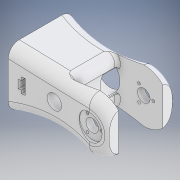
# Autodesk Inventor part: AA010
Saved by Autodesk Inventor 2017 SP1 (Build 210196100, 196)
## iProperties
Created: 2017-09-29
Part Number: AA010
Material: ABS Plastic
Document SubType Name: Modeling
Designer: Zach
Density: 1.06 g/cm^3
Appearance: CR White
Author: Zach
Autodesk Inventor part; units mm, degrees
sketch "Sketch1" plane through (0, 0, 0) normal (0, 0, 1) x (1, 0, 0)
  line L0 (0, 0) -> (0, 105)
  circle A0 centre (75, 52.5) radius 2.5
  circle A1 centre (145, 52.5) radius 11.25
  circle A2 centre (145, 52.5) radius 47.5 construction
  arc A3 (145, 5) -> (0, 0) centre (84.2999, -339.6962) ccw
  arc A4 (0, 105) -> (145, 100) centre (84.2999, 444.6962) ccw
  arc A5 (145, 5) -> (145, 100) centre (145, 52.5) ccw
  point P0 (0, 52.5)
  dimension "d0" = 105
  dimension "d1" = 5
  dimension "d2" = 22.5
  dimension "d3" = 70
  dimension "d4" = 95
  dimension "d5" = 145
  dimension "d6" = 350
  dimension "d7" = 350
  constraints: 8 point on circle, 6 centre point, 2 end point, 2 horizontal alignment, 2 vertical alignment, 1 coincident, 1 concentric, 1 midpoint, 1 vertical
  measures "d0" distance of L0.start L0.end
  measures "d1" diameter of A0
  measures "d2" diameter of A1
  measures "d3" distance of A1.centre A0.centre
  measures "d4" diameter of A2
  measures "d5" distance of point (0, 52.5) A2.centre
  measures "d6" radius of A3
  measures "d7" radius of A4
extrude "Extrusion1" add sketch "Sketch1" along normal blind 115
sketch "Sketch2" plane through (0, 0, 0) normal (0, 1, 0) x (-1, 0, 0)
  line L0 (0, 0) -> (-145, 0) projected
  arc A0 (0, 0) -> (-145, 0) centre (-72.5, -342.4087) ccw
  line L1 (-145, 115) -> (0, 115) projected
  arc A1 (-145, 115) -> (0, 115) centre (-72.5, 457.4087) ccw
  dimension "d10" = 350
  dimension "d11" = 350
  constraints: 4 point on circle, 2 centre point
  measures "d10" radius of A0
  measures "d11" radius of A1
extrude "Extrusion2" cut sketch "Sketch2" along normal through all
ref_plane "Work Plane1" through (0, 0, 57.5) normal (0, 0, 1) x (1, 0, 0)
sketch "Sketch3" plane through (0, 0, 57.5) normal (0, 0, 1) x (1, 0, 0)
  arc A0 (145, 41.25) -> (145, 63.75) centre (145, 52.5) ccw projected
  arc A1 (145, 41.25) -> (145, 63.75) centre (145, 52.5) ccw projected
  circle A2 centre (145, 52.5) radius 52.5
  point P0 (0, 0)
  dimension "d15" = 105
  constraints: 1 centre point, 1 coincident
  measures "d15" diameter of A2
extrude "Extrusion3" cut sketch "Sketch3" along normal mid plane 79
fillet "Fillet2" radius 15 2 edges at (115.7763, 96.1145, 57.5) (115.7763, 8.8855, 57.5)
fillet "Fillet3" radius 20 4 edges at (71.9844, 94.913, 7.5909) (71.9844, 94.913, 107.4091) (71.9843, 10.087, 107.4091) (71.9843, 10.087, 7.5909)
fillet "Fillet4" radius 20 2 edges at (192.5, 52.5, 115) (192.5, 52.5, 0)
sketch "Sketch4" plane through (0, 19.5779, 115) normal (-1, 0, 0) x (0, 0, 1)
  line L0 (-72, 12.9221) -> (-97, 12.9221)
  line L1 (-97, 12.9221) -> (-97, 52.9221)
  line L2 (-97, 52.9221) -> (-72, 52.9221)
  line L3 (-72, 52.9221) -> (-72, 12.9221)
  line L4 (-95.5772, -19.5779) -> (-19.4228, -19.5779) projected
  line L5 (-115, 0) -> (-115, 65.8443) projected
  line L6 (-97, -14.5765) -> (-97, -7.145) projected
  line L7 (-97, 80.4208) -> (-97, -14.5765) projected
  line L8 (-97, 72.9893) -> (-97, 80.4208) projected
  line L9 (-97, 54.076) -> (-97, 72.9893) projected
  line L10 (-97, 11.7683) -> (-97, 54.076) projected
  line L11 (-97, -7.145) -> (-97, 11.7683) projected
  line L12 (-97, 21.6721) -> (-97, 44.1721) projected
  line L13 (-18, 44.1721) -> (-18, 21.6721) projected
  line L14 (-18, -7.145) -> (-18, -14.5765) projected
  line L15 (-18, 11.7683) -> (-18, -7.145) projected
  line L16 (-18, 54.076) -> (-18, 11.7683) projected
  line L17 (-18, 72.9893) -> (-18, 54.076) projected
  line L18 (-18, 80.4208) -> (-18, 72.9893) projected
  line L19 (-18, -14.5765) -> (-18, 80.4208) projected
  point P0 (-115, -19.5779)
  point P1 (-84.5, 12.9221)
  point P2 (-57.5, -19.5779)
  point P3 (-97, 32.9221)
  point P4 (-115, 32.9221)
  dimension "d21" = 25
  dimension "d22" = 40
  constraints: 8 end point, 5 midpoint, 2 parallel, 1 horizontal, 1 horizontal alignment, 1 perpendicular
  measures "d21" distance of L1.end L2.end
  measures "d22" distance of L0.end L1.end
extrude "Extrusion4" cut sketch "Sketch4" against normal through all
sketch "Sketch6" plane through (0, 0, 0) normal (0, 0, -1) x (-1, 0, 0)
  circle A0 centre (-145, 52.5) radius 22.5
  arc A1 (-145, 63.75) -> (-145, 41.25) centre (-145, 52.5) ccw projected
  point P0 (0, 0)
  dimension "d28" = 45
  constraints: 1 centre point, 1 concentric
  measures "d28" diameter of A0
extrude "Extrusion6" cut sketch "Sketch6" against normal blind 5
sketch "Sketch7" plane through (0, 0, 115) normal (0, 0, 1) x (1, 0, 0)
  circle A0 centre (145, 52.5) radius 22.5
  arc A1 (145, 41.25) -> (145, 63.75) centre (145, 52.5) ccw projected
  point P0 (0, 0)
  dimension "d31" = 45
  constraints: 1 centre point, 1 concentric
  measures "d31" diameter of A0
extrude "Extrusion7" cut sketch "Sketch7" against normal blind 5
sketch "Sketch8" plane through (145, 52.5, 110) normal (0, 0, 1) x (1, 0, 0)
  circle A0 centre (17, 0) radius 2.5
  circle A1 centre (0, 0) radius 11.25 construction
  circle A2 centre (-8.5, 14.7224) radius 2.5
  circle A3 centre (-8.5, -14.7224) radius 2.5
  point P0 (-145, -52.5)
  dimension "d34" = 5
  dimension "d35" = 17
  dimension "d38" = 360
  constraints: 3 centre point, 1 horizontal alignment, 7 other
  measures "d34" diameter of A0
  measures "d35" distance of A0.centre A1.centre
extrude "Extrusion8" cut sketch "Sketch8" against normal through all
sketch "Sketch47" plane through (0, 0, 18) normal (0, 0, 1) x (1, 0, 0)
  circle A0 centre (75, 52.5) radius 13
  spline S0 degree 2 poles (77.5, 52.5) (77.5, 48.1699) (73.75, 50.3349) (70, 52.5) (73.75, 54.6651) (77.5, 56.8301) (77.5, 52.5) knots 0 0 0 0.333333 0.333333 0.666667 0.666667 1 1 1 weights 1 0.5 1 0.5 1 0.5 1 projected
  circle A1 centre (75, 52.5) radius 2.5 projected
  point P0 (0, 0)
  dimension "d180" = 26
  constraints: 1 centre point, 1 coincident, 1 horizontal alignment, 1 other
  measures "d180" diameter of A0
extrude "Extrusion44" cut sketch "Sketch47" along normal through all
sketch "Sketch48" plane through (0, 32.5, 43) normal (0, 0, -1) x (-1, 0, 0)
  circle A0 centre (-75, 20) radius 2
  circle A1 centre (-66.5, 20) radius 2
  circle A2 centre (-83.5, 20) radius 2
  circle A3 centre (-75, 20) radius 13 projected
  line L0 (-83.5, 20) -> (-66.5, 20) construction
  point P0 (0, -32.5)
  dimension "d183" = 4
  dimension "d184" = 4
  dimension "d185" = 4
  dimension "d186" = 17
  constraints: 3 centre point, 2 coincident, 2 end point, 1 horizontal, 1 horizontal alignment, 1 midpoint, 1 other
  measures "d183" diameter of A0
  measures "d184" diameter of A1
  measures "d185" diameter of A2
  measures "d186" distance of L0.start L0.end
extrude "Extrusion45" add sketch "Sketch48" against normal blind 5
sketch "Sketch49" plane through (75, 52.5, 48) normal (0, 0, 1) x (1, 0, 0)
  circle A0 centre (0, 0) radius 2 projected
  circle A1 centre (0, 0) radius 3.5
  point P0 (-75, -52.5)
  dimension "d189" = 7
  constraints: 1 centre point, 1 coincident
  measures "d189" diameter of A1
extrude "Extrusion46" cut sketch "Sketch49" against normal blind 3
sketch "Sketch50" plane through (0, 32.5, 43) normal (0, 0, -1) x (-1, 0, 0)
  circle A0 centre (-83.5, 20) radius 2 projected
  circle A1 centre (-66.5, 20) radius 2 projected
  circle A2 centre (-83.5, 20) radius 3.5
  circle A3 centre (-66.5, 20) radius 3.5
  point P0 (0, -32.5)
  dimension "d192" = 7
  dimension "d193" = 7
  constraints: 2 centre point, 2 coincident
  measures "d192" diameter of A2
  measures "d193" diameter of A3
extrude "Extrusion47" cut sketch "Sketch50" against normal blind 3 contours A0 | A1 | A2 | A3
sketch "Sketch51" plane through (0, 0, 18) normal (0, 0, 1) x (1, 0, 0)
  circle A0 centre (75, 52.5) radius 2 projected
  circle A1 centre (75, 52.5) radius 27.5
  point P0 (0, 0)
  dimension "d196" = 55
  constraints: 1 centre point, 1 coincident
  measures "d196" diameter of A1
extrude "Extrusion48" cut sketch "Sketch51" against normal blind 15 and the other way blind 25
sketch "Sketch52" plane through (0, 19.5779, 115) normal (-1, 0, 0) x (0, 0, 1)
  circle A0 centre (-57.5, 32.9221) radius 4.25
  line L0 (-95.5772, -19.5779) -> (-19.4228, -19.5779) projected
  line L1 (-115, 0) -> (-115, 65.8443) projected
  point P0 (-115, -19.5779)
  point P1 (-57.5, -19.5779)
  point P2 (-115, 32.9221)
  dimension "d199" = 8.5
  constraints: 2 midpoint, 1 centre point, 1 horizontal alignment, 1 vertical alignment
  measures "d199" diameter of A0
extrude "Extrusion49" cut sketch "Sketch52" against normal blind 55
ref_plane "Work Plane7" through (0, 52.5, 115) normal (0, 0, 1) x (1, 0, 0)
sketch "Sketch55" plane through (0, 52.5, 115) normal (0, 0, 1) x (1, 0, 0)
  line L0 (26, -13) -> (20, -13)
  line L1 (20, -13) -> (20, 13)
  line L2 (20, 13) -> (26, 13)
  line L3 (26, 13) -> (26, -13)
  line L4 (20, -45) -> (20, 45)
  line L5 (26, -7.5) -> (15, -7.5)
  line L6 (15, -7.5) -> (15, 7.5)
  line L7 (15, 7.5) -> (26, 7.5)
  line L8 (26, 7.5) -> (26, -7.5)
  line L9 (0, -32.9221) -> (0, 32.9221) projected
  point P0 (20, 0)
  point P1 (15, 0)
  point P2 (0, 0)
  dimension "d203" = 6
  dimension "d204" = 26
  dimension "d218" = 11
  dimension "d219" = 15
  dimension "d231" = 20
  constraints: 18 end point, 4 midpoint, 4 parallel, 2 horizontal, 2 horizontal alignment, 2 perpendicular, 2 point on line
  measures "d203" distance of L1.end L2.end
  measures "d204" distance of L0.end L1.end
  measures "d218" distance of L6.end L7.end
  measures "d219" distance of L5.end L6.end
  measures "d231" distance between parallel lines of L1 L9
extrude "Extrusion50" cut sketch "Sketch55" against normal blind 72
sketch "Sketch56" plane through (26, 39.5, 110.5114) normal (-1, 0, 0) x (0, 0, 1)
  circle A0 centre (-53.0114, 22.525) radius 1.5
  circle A1 centre (-61.2603, 17.7625) radius 1.5
  circle A2 centre (-61.2603, 8.2375) radius 1.5
  circle A3 centre (-53.0114, 3.475) radius 1.5
  circle A4 centre (-44.7625, 8.2375) radius 1.5
  circle A5 centre (-44.7625, 17.7625) radius 1.5
  circle A6 centre (-53.0114, 13) radius 4.25 projected
  point P0 (111.3686, -39.5)
  point P1 (-53.0114, 13)
  dimension "d210" = 3
  dimension "d211" = 9.525
  dimension "d214" = 360
  constraints: 6 centre point, 1 coincident, 1 vertical alignment, 13 other
  measures "d210" diameter of A0
  measures "d211" distance of point (-53.011, 13) A0.centre
extrude "Extrusion51" cut sketch "Sketch56" against normal blind 20 contours A0 | A1 | A2 | A3 | A4 | A5
sketch "Sketch58" plane through (26, 39.5, 110.5114) normal (-1, 0, 0) x (0, 0, 1)
  circle A0 centre (-53.0114, 3.475) radius 3.5
  circle A1 centre (-53.0114, 13) radius 4.5 construction
  circle A2 centre (-44.7625, 8.2375) radius 3.5
  circle A3 centre (-44.7625, 17.7625) radius 3.5
  circle A4 centre (-53.0114, 22.525) radius 3.5
  circle A5 centre (-61.2603, 17.7625) radius 3.5
  circle A6 centre (-61.2603, 8.2375) radius 3.5
  circle A7 centre (-53.0114, 3.475) radius 1.5 construction
  circle A8 centre (-53.0114, 13) radius 4.25 construction
  point P0 (-115, -19.5779)
  dimension "d220" = 7
  dimension "d223" = 360
  constraints: 7 centre point, 2 coincident, 1 vertical alignment, 14 other
  measures "d220" diameter of A0
extrude "Extrusion52" cut sketch "Sketch58" along normal through all
sketch "Sketch59" plane through (0, 19.5779, 115) normal (-1, 0, 0) x (0, 0, 1)
  line L0 (-97, 12.9221) -> (-97, 52.9221) projected
  line L1 (-72, 12.9221) -> (-97, 12.9221) projected
  line L2 (-72, 52.9221) -> (-72, 12.9221) projected
  line L3 (-97, 52.9221) -> (-72, 52.9221) projected
  point P0 (-115, -19.5779)
extrude "Extrusion53" add sketch "Sketch59" against normal blind 35
ref_plane "Work Plane8" through (179, 19.5779, 115) normal (-1, 0, 0) x (0, 0, 1)
fillet "Fillet5" radius 5 7 edges at (96.7011, 73.0784, 18) (97.6664, 83.7422, 18) (96.7011, 31.9216, 18) (97.6664, 21.2578, 18) (92.5, 52.5, 97) (97.6664, 21.2578, 97) (97.6664, 83.7422, 97)
sketch "Sketch64" plane through (145, 52.5, 43) normal (0, 0, -1) x (-1, 0, 0)
  line L0 (110, -20) -> (110, 20) projected
  line L1 (110, 20) -> (88.8746, 20) projected
  line L2 (110, -20) -> (88.8746, -20) projected
  arc A0 (88.8746, -20) -> (88.8746, 20) centre (70, 0) ccw
  circle A1 centre (70, 0) radius 2 projected
  point P0 (145, -52.5)
  constraints: 2 point on circle, 1 centre point, 1 coincident, 1 vertical alignment
extrude "Extrusion55" add sketch "Sketch64" along normal blind 25 contours L2 A0 L1 L0
sketch "Sketch63" plane through (179, 19.5779, 115) normal (-1, 0, 0) x (0, 0, 1)
  circle A0 centre (-65.7489, 37.6846) radius 3.5 projected
  circle A1 centre (-49.2511, 37.6846) radius 3.5 projected
  circle A2 centre (-57.5, 23.3971) radius 3.5 projected
  circle A3 centre (-49.2511, 28.1596) radius 3.5 projected
  circle A4 centre (-57.5, 42.4471) radius 3.5 projected
  circle A5 centre (-65.7489, 28.1596) radius 3.5 projected
  circle A6 centre (-57.5, 32.9221) radius 4.25 projected
  spline S0 degree 6 poles (-95.5772, -19.5779) (-95.5791, -19.5779) (-95.581, -19.5779) (-95.5829, -19.5779) (-95.5848, -19.5779) (-96.4358, -19.5777) (-97.2903, -19.5343) (-98.1439, -19.4475) (-98.9955, -19.316) (-99.842, -19.1393) (-101.133, -18.7972) (-101.5834, -18.6638) (-102.0309, -18.5172) (-102.4748, -18.3572) (-102.9145, -18.184) (-104.2495, -17.6121) (-105.1293, -17.1701) (-105.9834, -16.6728) (-106.8065, -16.122) (-107.5936, -15.5207) (-108.9202, -14.3691) (-109.476, -13.8373) (-110.0052, -13.2791) (-110.506, -12.6966) (-110.977, -12.0921) (-111.6183, -11.1828) (-111.813, -10.8934) (-112.0012, -10.6002) (-112.1827, -10.3033) (-112.3576, -10.003) (-112.7996, -9.2046) (-113.0557, -8.7012) (-113.2935, -8.1903) (-113.5129, -7.6729) (-113.7139, -7.1498) (-114.2685, -5.5467) (-114.5641, -4.4517) (-114.7834, -3.3445) (-114.9281, -2.2297) (-114.9999, -1.1152) (-115, -0.0059) (-115, -0.0039) (-115, -0.002) (-115, 0) knots 0 0 0 0 0 0 0 0.000376 0.000376 0.000376 0.000376 0.1699 0.1699 0.1699 0.1699 0.1699 0.261533 0.261533 0.261533 0.261533 0.261533 0.451167 0.451167 0.451167 0.451167 0.451167 0.598573 0.598573 0.598573 0.598573 0.598573 0.66595 0.66595 0.66595 0.66595 0.66595 0.775808 0.775808 0.775808 0.775808 0.775808 0.999604 0.999604 0.999604 1 1 1 1 1 1 1 projected
  line L0 (-95.5772, -19.5779) -> (-19.4228, -19.5779) projected
  spline S1 degree 6 poles (0, 0) (0, -0.002) (0, -0.0039) (0, -0.0059) (-0.0001, -1.1152) (-0.0719, -2.2297) (-0.2166, -3.3445) (-0.4359, -4.4517) (-0.7315, -5.5467) (-1.2861, -7.1498) (-1.4871, -7.6729) (-1.7065, -8.1903) (-1.9443, -8.7012) (-2.2004, -9.2046) (-2.6424, -10.003) (-2.8173, -10.3033) (-2.9988, -10.6002) (-3.187, -10.8934) (-3.3817, -11.1828) (-4.023, -12.0921) (-4.494, -12.6966) (-4.9948, -13.2791) (-5.524, -13.8373) (-6.0798, -14.3691) (-7.4064, -15.5207) (-8.1935, -16.122) (-9.0166, -16.6728) (-9.8707, -17.1701) (-10.7505, -17.6121) (-12.0855, -18.184) (-12.5252, -18.3572) (-12.9691, -18.5172) (-13.4166, -18.6638) (-13.867, -18.7972) (-15.158, -19.1393) (-16.0045, -19.316) (-16.8561, -19.4475) (-17.7097, -19.5343) (-18.5642, -19.5777) (-19.4152, -19.5779) (-19.4171, -19.5779) (-19.419, -19.5779) (-19.4209, -19.5779) (-19.4228, -19.5779) knots 0 0 0 0 0 0 0 0.000396 0.000396 0.000396 0.224192 0.224192 0.224192 0.224192 0.224192 0.33405 0.33405 0.33405 0.33405 0.33405 0.401427 0.401427 0.401427 0.401427 0.401427 0.548833 0.548833 0.548833 0.548833 0.548833 0.738467 0.738467 0.738467 0.738467 0.738467 0.8301 0.8301 0.8301 0.8301 0.8301 0.999624 0.999624 0.999624 0.999624 1 1 1 1 1 1 1 projected
  line L1 (0, 65.8443) -> (0, 0) projected
  spline S2 degree 6 poles (-19.4228, 85.4221) (-19.4209, 85.4221) (-19.419, 85.4221) (-19.4171, 85.4221) (-18.5673, 85.4221) (-17.714, 85.3789) (-16.8598, 85.2921) (-16.0095, 85.161) (-15.1641, 84.9849) (-13.8709, 84.6426) (-13.4171, 84.5084) (-12.9664, 84.3606) (-12.5193, 84.1994) (-12.0764, 84.0247) (-10.74, 83.4511) (-9.8618, 83.0092) (-9.0093, 82.5123) (-8.1877, 81.9621) (-7.4021, 81.3615) (-6.079, 80.2126) (-5.5254, 79.6827) (-4.9982, 79.1267) (-4.4991, 78.5466) (-4.0295, 77.9447) (-3.3882, 77.0367) (-3.1923, 76.746) (-3.0031, 76.4513) (-2.8205, 76.153) (-2.6447, 75.8513) (-2.2034, 75.0545) (-1.9487, 74.5543) (-1.7121, 74.0467) (-1.4936, 73.5326) (-1.2933, 73.0129) (-0.7366, 71.4098) (-0.439, 70.3112) (-0.2181, 69.2003) (-0.0726, 68.0836) (-0.0003, 66.9652) (0, 65.8521) (0, 65.8501) (0, 65.8482) (0, 65.8462) (0, 65.8443) knots 0 0 0 0 0 0 0 0.000376 0.000376 0.000376 0.169655 0.169655 0.169655 0.169655 0.169655 0.261961 0.261961 0.261961 0.261961 0.261961 0.451294 0.451294 0.451294 0.451294 0.451294 0.598143 0.598143 0.598143 0.598143 0.598143 0.665855 0.665855 0.665855 0.665855 0.665855 0.775036 0.775036 0.775036 0.775036 0.775036 0.999604 0.999604 0.999604 0.999604 1 1 1 1 1 1 1 projected
  line L2 (-95.5772, 85.4221) -> (-19.4228, 85.4221) projected
  spline S3 degree 6 poles (-115, 65.8443) (-115, 65.8462) (-115, 65.8482) (-115, 65.8501) (-115, 65.8521) (-114.9997, 66.9652) (-114.9274, 68.0836) (-114.7819, 69.2003) (-114.561, 70.3112) (-114.2634, 71.4098) (-113.7067, 73.0129) (-113.5064, 73.5326) (-113.2879, 74.0467) (-113.0513, 74.5543) (-112.7966, 75.0545) (-112.3553, 75.8513) (-112.1795, 76.153) (-111.9969, 76.4513) (-111.8077, 76.746) (-111.6118, 77.0367) (-110.9705, 77.9447) (-110.5009, 78.5466) (-110.0018, 79.1267) (-109.4746, 79.6827) (-108.921, 80.2126) (-107.5979, 81.3615) (-106.8123, 81.9621) (-105.9907, 82.5123) (-105.1382, 83.0092) (-104.26, 83.4511) (-102.9236, 84.0247) (-102.4807, 84.1994) (-102.0336, 84.3606) (-101.5829, 84.5084) (-101.1291, 84.6426) (-99.8359, 84.9849) (-98.9905, 85.161) (-98.1402, 85.2921) (-97.286, 85.3789) (-96.4327, 85.4221) (-95.5829, 85.4221) (-95.581, 85.4221) (-95.5791, 85.4221) (-95.5772, 85.4221) knots 0 0 0 0 0 0 0 0.000396 0.000396 0.000396 0.000396 0.224964 0.224964 0.224964 0.224964 0.224964 0.334145 0.334145 0.334145 0.334145 0.334145 0.401857 0.401857 0.401857 0.401857 0.401857 0.548706 0.548706 0.548706 0.548706 0.548706 0.738039 0.738039 0.738039 0.738039 0.738039 0.830345 0.830345 0.830345 0.830345 0.830345 0.999624 0.999624 0.999624 1 1 1 1 1 1 1 projected
  line L3 (-115, 0) -> (-115, 65.8443) projected
  point P0 (-115, -19.5779)
  constraints: 4 other
extrude "Extrusion54" cut sketch "Sketch63" against normal through all
body "Solid1"
